Autodesk Fusion 360 part; units mm, degrees
note: some values were not read from the file. Chosen so that the rebuilt part matches the saved one: which face or edge a step refers to; which pieces of a blend or face edit are solid. Set by a fixed rule: which sketch regions a step uses; the direction of a hole.
(part 2 of 2)
sketch "Sketch22" plane through (0, 0, 3.25) normal (0, 0, 1) x (-1, 0, 0)
  line L0 (-66.04, -14.41) -> (-63.86, -14.41)
  arc A0 (-63.86, -18.41) -> (-63.86, -14.41) centre (-63.86, -16.41) ccw
  line L1 (-63.86, -18.41) -> (-66.04, -18.41)
  line L2 (-66.04, -18.41) -> (-66.04, -23.4)
  arc A1 (-66.04, -23.4) -> (-64.04, -25.4) centre (-64.04, -23.4) ccw
  line L3 (-64.04, -25.4) -> (-19.62, -25.4)
  line L4 (-19.62, -25.4) -> (-19.62, -27.4)
  line L5 (-19.62, -27.4) -> (-14.32, -27.4)
  line L6 (-14.32, -27.4) -> (-14.32, -25.4)
  line L7 (-14.32, -25.4) -> (-2, -25.4)
  arc A2 (-2, -25.4) -> (0, -23.4) centre (-2, -23.4) ccw
  line L8 (0, -23.4) -> (0, -19.3644)
  circle A3 centre (-1.5, -19.3644) radius 1.5
  line L9 (0, -19.3644) -> (0, -16.08)
  line L10 (0, -16.08) -> (1.75, -16.08)
  line L11 (1.75, -16.08) -> (1.75, -9.08)
  line L12 (1.75, -9.08) -> (0, -9.08)
  line L13 (0, -9.08) -> (0, -2)
  arc A4 (0, -2) -> (-2, 0) centre (-2, -2) ccw
  line L14 (-2, 0) -> (-5.99, 0)
  line L15 (-5.99, 0) -> (-5.99, 2)
  line L16 (-5.99, 2) -> (-12.99, 2)
  line L17 (-12.99, 2) -> (-12.99, 0)
  line L18 (-12.99, 0) -> (-15.32, 0)
  line L19 (-15.32, 0) -> (-16.07, 0.75)
  line L20 (-16.07, 0.75) -> (-18.57, 0.75)
  line L21 (-18.57, 0.75) -> (-19.32, 0)
  line L22 (-19.32, 0) -> (-57.82, 0)
  line L23 (-57.82, 0) -> (-58.57, 0.75)
  line L24 (-58.57, 0.75) -> (-61.07, 0.75)
  line L25 (-61.07, 0.75) -> (-61.82, 0)
  line L26 (-61.82, 0) -> (-64.04, 0)
  arc A5 (-64.04, 0) -> (-66.04, -2) centre (-64.04, -2) ccw
  line L27 (-66.04, -2) -> (-66.04, -14.41)
  line L28 (-19.07, -0.37) -> (-19.07, -4.77)
  line L29 (-19.07, -4.77) -> (-58.07, -4.77)
  line L30 (-58.07, -4.77) -> (-58.07, -0.37)
  line L31 (-58.07, -0.37) -> (-19.07, -0.37)
  circle A6 centre (-64.01, -2.03) radius 1.125
  circle A7 centre (-2.03, -23.37) radius 1.125
  circle A8 centre (-64.01, -23.37) radius 1.125
  circle A9 centre (-2.03, -2.03) radius 1.125
  line L32 (-13.09, -7.91) -> (-13.09, -17.91)
  line L33 (-13.09, -17.91) -> (-23.09, -17.91)
  line L34 (-23.09, -17.91) -> (-23.09, -7.91)
  line L35 (-23.09, -7.91) -> (-13.09, -7.91)
  line L36 (-58.07, -25.03) -> (-58.07, -20.63)
  line L37 (-58.07, -20.63) -> (-19.07, -20.63)
  line L38 (-19.07, -20.63) -> (-19.07, -25.03)
  line L39 (-19.07, -25.03) -> (-58.07, -25.03)
  circle A10 centre (-2.25, -6.1356) radius 1.5
  line L40 (-64.29, -11.41) -> (-59.29, -11.41)
  line L41 (-59.29, -11.41) -> (-59.29, -4.61)
  line L42 (-59.29, -4.61) -> (-64.29, -4.61)
  line L43 (-64.29, -4.61) -> (-64.29, -11.41)
  dimension "d356" = 5
  dimension "d357" = 6.8
  dimension "d358" = 1.75
  dimension "d359" = 3
  constraint horizontal L40
  constraint vertical L41
  constraint horizontal L42
  constraint vertical L43
  measures "d356" distance of L40.start L40.end
  measures "d357" distance of L40.end L41.end
  measures "d358" distance of L27 L43
  measures "d359" distance of L0 L40
extrude "Extrude34" add sketch "Sketch22" along normal blind 2 draft -20 contours L40 L41 L42 L43 bodies 1
chamfer "Chamfer14" distance 1 angle 45 13 edges at (-3, 12.58, 17.8) (69.04, 11.635, 17.8) (69.04, 16.52, 16.3) (33.02, -3, 17.8) (-1.9749, -1.9749, 17.8) (-3, 4.29, 17.8) (69.04, 4.125, 17.8) (68.0149, -1.9749, 17.8) (33.02, 28.4, 17.8) (68.0149, 27.3749, 17.8) (69.04, 23.21, 17.8) (-3, 20.99, 17.8) (-1.9749, 27.3749, 17.8) on bodies 1 4
chamfer "Chamfer14" distance 1 angle 45 4 edges at (18.09, 17.91, 3.25) (13.09, 12.91, 3.25) (23.09, 12.91, 3.25) (18.09, 7.91, 3.25) on bodies 1 4
sketch "Sketch23" plane through (0, -3, 0) normal (0, -1, 0) x (1, 0, 0)
  line L0 (33.58, 7.95) -> (22.55, 7.95)
  arc A0 (21.05, 9.45) -> (22.55, 7.95) centre (22.55, 9.45) ccw
  line L1 (21.05, 9.45) -> (21.05, 11.25)
  arc A1 (22.55, 12.75) -> (21.05, 11.25) centre (22.55, 11.25) ccw
  line L2 (22.55, 12.75) -> (33.58, 12.75)
  arc A2 (35.08, 11.25) -> (33.58, 12.75) centre (33.58, 11.25) ccw
  line L3 (35.08, 11.25) -> (35.08, 9.45)
  arc A3 (33.58, 7.95) -> (35.08, 9.45) centre (33.58, 9.45) ccw
  circle A4 centre (22.6, 4) radius 3
  circle A5 centre (57.1, 4) radius 3
  line L4 (13.99, 2.25) -> (4.99, 2.25)
  line L5 (4.99, 2.25) -> (4.99, 7.45)
  line L6 (4.99, 7.45) -> (13.99, 7.45)
  line L7 (13.99, 7.45) -> (13.99, 2.25)
  line L8 (65.54, 16.8) -> (0.5, 16.8)
  line L9 (0.5, 16.8) -> (0.5, 1)
  line L10 (0.5, 1) -> (14.6, 1)
  line L11 (14.6, 1) -> (15.6, 0)
  line L12 (15.6, 0) -> (64.1, 0)
  line L13 (64.1, 0) -> (65.1, 1)
  line L14 (65.1, 1) -> (65.54, 1)
  line L15 (65.54, 1) -> (65.54, 16.8)
  line L16 (69.04, 1) -> (69.04, 16.8)
  line L17 (-3, 16.8) -> (-3, 1)
  circle A6 centre (22.6, 4) radius 3
  circle A7 centre (57.1, 4) radius 3
  line L18 (39.85, 13.1866) -> (39.85, 3.1866) construction
  line L19 (33.02, 13.4639) -> (33.02, 3.4639) construction
  dimension "d374" = 10
  dimension "d375" = 10
  constraint vertical L18
  constraint vertical L19
  constraint symmetric A4.centre A5.centre L18
  constraint symmetric L16 L17 L19
  measures "d374" distance of L18.start L18.end
  measures "d375" distance of L19.start L19.end
equation "d6 = d4"
equation "d7 = d5"
equation "d16 = d18"
equation "d17 = d18"
equation "d18 = 1 mm"
equation "d19 = d18"
equation "d30 = d31"
equation "d31 = 3 mm + 1.75 mm"
equation "d45 = d46"
equation "d47 = d46"
equation "d48 = d46"
equation "d205 = d204"
equation "d211 = d210"
equation "d213 = d212"
equation "d215 = 50.5 mm - 16 mm"
equation "d259 = d258"
equation "d312 = 11.56 mm + 0.5 mm"
equation "d324 = 5.75 mm + ( ( 5 / 2 ) * 1 mm )"
equation "d325 = 1.5 mm + ( d326 / 3 ) + 0.5 mm"
equation "d336 = 3.2 mm + 5 mm - 1 mm - 2 mm"
equation "d338 = d337"
equation "d339 = 1.8 mm + 2 mm"
